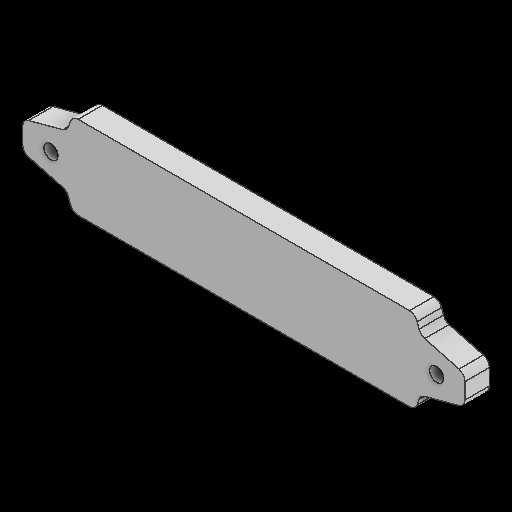
# Autodesk Inventor part: BatteryMount
Saved by Autodesk Inventor 2025.2 (Build 292293000, 293)
## iProperties
Created: 2026-05-27
Part Number: BatteryMount
Material: Generic
Document SubType Name: Modeling
Designer: valer
Density: 1 g/cm^3
Appearance: Default
Author: valer
Autodesk Inventor part; units mm, degrees
ref_plane "YZ Plane" through (0, 0, 0) normal (1, 0, 0) x (0, 1, 0)
ref_plane "XZ Plane" through (0, 0, 0) normal (0, 1, 0) x (-1, 0, 0)
ref_plane "XY Plane" through (0, 0, 0) normal (0, 0, 1) x (1, 0, 0)
sketch "Base" plane through (0, 0, 0) normal (0, 0, 1) x (1, 0, 0)
  line L0 (-152.6, 0) -> (152.6, 0) construction
  line L1 (0, -28.7) -> (0, 28.7) construction
  circle A0 centre (-95, 0) radius 3.5
  circle A1 centre (95, 0) radius 3.5
  line L2 (-109, 7) -> (-109, 0)
  line L3 (-109, 7) -> (-87.0124, 12.8915)
  line L4 (-87.0124, 12.8915) -> (-84.5403, 20.5)
  line L5 (-84.5403, 20.5) -> (0, 20.5)
  line L6 (-109, -7) -> (-109, 0)
  line L7 (-109, -7) -> (-87.0124, -12.8915)
  line L8 (-87.0124, -12.8915) -> (-84.5403, -20.5)
  line L9 (-84.5403, -20.5) -> (0, -20.5)
  line L10 (109, 7) -> (109, 0)
  line L11 (109, 7) -> (87.0124, 12.8915)
  line L12 (87.0124, 12.8915) -> (84.5403, 20.5)
  line L13 (84.5403, 20.5) -> (0, 20.5)
  line L14 (84.5403, -20.5) -> (0, -20.5)
  line L15 (87.0124, -12.8915) -> (84.5403, -20.5)
  line L16 (109, -7) -> (87.0124, -12.8915)
  line L17 (109, -7) -> (109, 0)
  point P0 (0, 0)
  dimension "d0" = 7
  dimension "d1" = 190
  dimension "d3" = 108
  dimension "d4" = 165
  dimension "d5" = 8
  dimension "d6" = 7
  dimension "d7" = 218
  dimension "d8" = 41
  constraints: 32 end point, 12 symmetric about line, 3 point on line, 2 centre point, 1 perpendicular, 1 vertical, 1 other
  measures "d0" diameter of A0
  measures "d1" distance of A1.centre A0.centre
  measures "d3" angle of L5 L4
  measures "d4" angle of L5 L3
  measures "d5" distance of L3.end L4.end
  measures "d6" distance of L2.start L2.end
  measures "d7" distance between parallel lines of L10 L2
  measures "d8" distance between parallel lines of L9 L5
extrude "BaseFeature" add sketch "Base" along normal blind 12
fillet "OutsideFilletsFeature" radius 4 12 edges at (-109, -7, 6) (-109, 7, 6) (-87.0124, -12.8915, 6) (-84.5403, -20.5, 6) (-87.0124, 12.8915, 6) (-84.5403, 20.5, 6) (84.5403, 20.5, 6) (87.0124, 12.8915, 6) (109, -7, 6) (87.0124, -12.8915, 6) (84.5403, -20.5, 6) (109, 7, 6)
body "Solid1"
